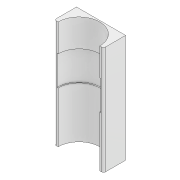
# Autodesk Inventor part: motor_support2
Saved by Autodesk Inventor 2020 (Build 240168000, 168)
## iProperties
Created: 2020-08-28
Part Number: motor_support2
Material: ABS 플라스틱
Document SubType Name: Modeling
Designer: 이호석
Mass: 150 g
Surface Area: 194.46 cm^2
Volume: 43.6486 cm^3
Density: 3.43654 g/cm^3
Appearance: 매끄러움 - 흰색
Author: 이호석
Autodesk Inventor part; units mm, degrees
ref_plane "YZ Plane" through (0, 0, 0) normal (1, 0, 0) x (0, 1, 0)
ref_plane "XZ Plane" through (0, 0, 0) normal (0, 1, 0) x (-1, 0, 0)
ref_plane "XY Plane" through (0, 0, 0) normal (0, 0, 1) x (1, 0, 0)
sketch "스케치1" plane through (0, 0, 0) normal (0, 0, 1) x (1, 0, 0)
  line L0 (-25, 55) -> (25, 55)
  line L1 (25, 55) -> (25, -55)
  line L2 (25, -55) -> (-25, -55)
  line L3 (-25, -55) -> (-25, 55)
  line L4 (-25, 55) -> (25, -55) construction
  line L5 (25, 55) -> (-25, -55) construction
  point P0 (0, 0)
  dimension "d0" = 50
  dimension "d1" = 110
  constraints: 12 end point, 2 midpoint, 2 parallel, 1 horizontal, 1 perpendicular
  measures "d0" distance of L1.end L2.end
  measures "d1" distance of L0.end L1.end
extrude "돌출1" add sketch "스케치1" along normal blind 41.5
sketch "스케치2" plane through (-25, -55, 0) normal (0, -1, 0) x (1, 0, 0)
  line L0 (50, 0) -> (0, 0) projected
  line L1 (0, 0) -> (25, 0)
  line L2 (25, 0) -> (25, 41.5)
  line L3 (50, 41.5) -> (0, 41.5) projected
  circle A0 centre (25, 41.5) radius 21.2
  dimension "d4" = 42.4
  constraints: 4 end point, 1 centre point, 1 coincident, 1 collinear, 1 midpoint
  measures "d4" diameter of A0
extrude "돌출2" cut sketch "스케치2" against normal blind 51.9
sketch "스케치3" plane through (-25, -3.1, 0) normal (0, -1, 0) x (1, 0, 0)
  line L0 (0, 0) -> (25, 0)
  line L1 (0, 0) -> (50, 0) projected
  line L2 (25, 0) -> (25, 41.5)
  line L3 (50, 41.5) -> (0, 41.5) projected
  circle A0 centre (25, 41.5) radius 22.3
  dimension "d7" = 44.6
  constraints: 4 end point, 1 centre point, 1 coincident, 1 collinear, 1 midpoint
  measures "d7" diameter of A0
extrude "돌출3" cut sketch "스케치3" against normal blind 30
sketch "스케치4" plane through (-25, 26.9, 0) normal (0, -1, 0) x (1, 0, 0)
  line L0 (50, 0) -> (0, 0)
  line L1 (0, 0) -> (25, 0)
  line L2 (25, 0) -> (25, 41.5)
  line L3 (50, 41.5) -> (0, 41.5)
  circle A0 centre (25, 41.5) radius 21.2
  dimension "d10" = 42.4
  constraints: 8 end point, 1 centre point, 1 coincident, 1 collinear, 1 midpoint
  measures "d10" diameter of A0
extrude "돌출4" cut sketch "스케치4" against normal through all
fillet "모깎기1" radius 2 2 edges at (-25, 0, 41.5) (25, 0, 41.5)
sketch "스케치5" plane through (-25, 55, 0) normal (0, 1, 0) x (1, 0, 0)
  arc A0 (47.3, -41.5) -> (2.7, -41.5) centre (25, -41.5) ccw projected
  arc A1 (47.3, -41.5) -> (2.7, -41.5) centre (25, -41.5) ccw projected
  line L0 (0, 0) -> (0, -39.5) projected
  line L1 (50, 0) -> (50, -39.5) projected
  line L2 (0, 0) -> (50, 0)
  line L3 (50, 0) -> (50, -19)
  line L4 (50, -19) -> (0, -19)
  line L5 (0, -19) -> (0, 0)
  point P0 (25, 0)
  dimension "d15" = 19
  constraints: 8 end point, 2 parallel, 1 horizontal, 1 perpendicular, 1 point on line
  measures "d15" distance of L2.end L3.end
extrude "돌출5" cut sketch "스케치5" against normal through all
